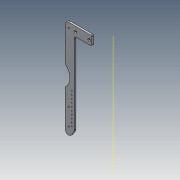
# Autodesk Inventor part: VP TRAY GUIDE SPLIT SHELF
Saved by Autodesk Inventor 2018.3 (Build 223284000, 284)
## iProperties
Created: 2018-09-09
Material: ACETAL COPOLYMER, WHITE
Vendor: HHMI: JRC - ID&F
Document SubType Name: Modeling
Designer: arnoldj
Density: 1.42 g/cm^3
Appearance: Plastic (White)
RuleStatus: InUse
AfterDocSave0: file://Part Number Cleaner
DESIGN DEPARTMENT: HHMI: JRC - ID&F
ALTERED ITEM PART NUMBER: N/A
ALTERED ITEM VENDOR: N/A
ALTERED ITEM DESCRIPTION: N/A
Author: arnoldj
Revision Number: 0
Autodesk Inventor part; units mm, degrees
ref_plane "YZ Plane" through (0, 0, 0) normal (1, 0, 0) x (0, 1, 0)
ref_plane "XZ Plane" through (0, 0, 0) normal (0, 1, 0) x (-1, 0, 0)
ref_plane "XY Plane" through (0, 0, 0) normal (0, 0, 1) x (1, 0, 0)
sketch "Sketch1" plane through (0, 0, 0) normal (0, 0, 1) x (1, 0, 0)
  line L0 (0, 251.46) -> (0, -264.16) projected
  line L1 (-361.3785, 0) -> (361.3785, 0) projected
  line L2 (177.8, -190.5) -> (-177.8, -190.5)
  line L3 (-177.8, -190.5) -> (-177.8, 177.8)
  line L4 (-177.8, 177.8) -> (177.8, 177.8)
  line L5 (177.8, 177.8) -> (177.8, -190.5)
  line L6 (143.51, -143.511) -> (-143.51, -143.511) construction
  line L7 (-143.51, -143.511) -> (-143.51, 143.509) construction
  line L8 (-143.51, 143.509) -> (143.51, 143.509) construction
  line L9 (143.51, 143.509) -> (143.51, -143.511) construction
  line L10 (-177.8, 177.8) -> (-177.8, 177.8)
  line L11 (-177.8, -190.5) -> (-177.8, 177.8)
  line L12 (177.8, 177.8) -> (177.8, 177.8)
  line L13 (177.8, -190.5) -> (177.8, 177.8)
  line L14 (-165.1, -158.75) -> (165.1, -158.75) construction
  line L15 (165.1, -158.75) -> (165.1, 158.75) construction
  line L16 (165.1, 158.75) -> (-165.1, 158.75) construction
  line L17 (-165.1, 158.75) -> (-165.1, -158.75) construction
  line L18 (144.4625, 143.509) -> (-144.4625, 143.509)
  line L19 (-144.4625, 143.509) -> (-144.4625, -190.5)
  line L20 (-144.4625, -190.5) -> (144.4625, -190.5)
  line L21 (144.4625, -190.5) -> (144.4625, 143.509)
  line L22 (144.4625, 143.509) -> (-144.4625, -190.5) construction
  line L23 (-144.4625, 143.509) -> (144.4625, -190.5) construction
  circle A0 centre (-209.55, 0) radius 48.5775
  circle A1 centre (209.55, 0) radius 48.5775
  line L24 (-65.455, 153.009) -> (-55.955, 153.009) construction
  line L25 (0, 177.8) -> (0, 143.509)
  point P0 (0, 0)
  point P1 (0, -23.4955)
  point P2 (-71.755, 153.009)
  point P3 (-139.7, 158.75)
  point P4 (139.7, 158.75)
  point P5 (0, 158.75)
  point P6 (-88.9, 158.75)
  point P7 (88.9, 158.75)
  point P8 (-165.1, -95.25)
  point P9 (165.1, -95.25)
  dimension "d2" = 355.6
  dimension "d66" = 177.8
  dimension "d70" = 368.3
  dimension "d71" = 177.8
  dimension "d85" = 287.02
  dimension "d86" = 330.2
  dimension "d94" = 288.925
  dimension "d95" = 0
  dimension "d107" = 209.55
  dimension "d108" = 97.155
  dimension "d111" = 209.55
  dimension "d112" = 9.5
  dimension "d113" = 9.5
  dimension "d115" = 15.8
  dimension "d116" = 71.755
  dimension "d124" = 139.7
  dimension "d125" = 139.7
  dimension "d133" = 317.5
  dimension "d134" = 165.1
  dimension "d135" = 158.75
  dimension "d136" = 50.8
  dimension "d137" = 50.8
  dimension "d158" = 63.5
  dimension "d159" = 63.5
  dimension "d160" = 55.955
  constraints: 48 end point, 12 point on line, 7 horizontal, 7 parallel, 5 coincident, 5 midpoint, 5 perpendicular, 2 centre point, 2 horizontal alignment, 1 equal radius
  measures "d2" distance of L3.end L4.end
  measures "d66" distance between parallel lines of L0 L3
  measures "d70" distance of L2.end L3.end
  measures "d71" distance between parallel lines of L1 L4
  measures "d85" distance of L6.end L7.end
  measures "d86" distance of L15.end L16.end
  measures "d94" distance of L18.start L18.end
  measures "d95" distance between parallel lines of L18 L8
  measures "d107" distance from line of L0 A0.centre
  measures "d108" diameter of A0
  measures "d111" distance from line of L0 A1.centre
  measures "d112" distance of L24.start L24.end
  measures "d113" distance between parallel lines of L24 L8
  measures "d115" distance of point (-55.955, 153.009) point (-71.755, 153.009)
  measures "d116" distance from line of L0 point (-71.755, 153.009)
  measures "d124" distance from line of point (-139.7, 158.75) L0
  measures "d125" distance from line of L0 point (139.7, 158.75)
  measures "d133" distance of L16.end L14.start
  measures "d134" distance between parallel lines of L0 L17
  measures "d135" distance between parallel lines of L1 L16
  measures "d136" distance of point (-139.7, 158.75) point (-88.9, 158.75)
  measures "d137" distance of point (88.9, 158.75) point (139.7, 158.75)
  measures "d158" distance from line of L14 point (-165.1, -95.25)
  measures "d159" distance of point (165.1, -95.25) point (165.1, -158.75)
  measures "d160" distance from line of L0 L24.end
extrude "Extrusion1" add sketch "Sketch1" against normal blind 6.35 contours L4 L5 A1 L1 L21 L18 L0 | L0 L18 L19 L1 A0 L3 L4 | L18 L21 L1 L0 | L0 L1 L19 L18 | L1 L21 L2 L0 | L0 L2 L19 L1 | A0 L1 L3 | L5 L1 A1 | L19 L2 L3 A0 L1 | L1 A1 L5 L2 L21 | L1 A0 L3 | L5 A1 L1 picked at (-175.8618, 22.522) picked at (175.8618, 22.522) picked at (-175.8618, -22.522) picked at (175.8618, -22.522)
hole "Hole5" at (-165.1, 158.75, 0) at (165.1, 158.75, 0) at (165.1, -158.75, 0) at (-165.1, -158.75, 0) at (-165.1, -95.25, 0) at (165.1, -95.25, 0) direction (0, 0, -1) diameter 5.1054 end through all clearance for "Flat Head Machine Screw (82)" size "#10" standard "Ansi Unified Screw Threads"
extrude "Extrusion5" cut sketch "Sketch1" against normal up to next contours L18 L21 L1 L0 | L0 L1 L19 L18 | L1 L21 L2 L0 | L0 L2 L19 L1
chamfer "Chamfer3" distance 15.875 angle 60 1 edges at (-144.4625, -190.5, -3.175) measured on face at (-166.6875, -190.5, -4.2333)
chamfer "Chamfer4" distance 15.875 angle 60 1 edges at (144.4625, -190.5, -3.175) measured on face at (155.575, -190.5, -4.2333)
fillet "Fillet8" radius 12.7 4 edges at (160.3375, -190.5, -3.175) (144.4625, -163.0037, -3.175) (-144.4625, -163.0037, -3.175) (-160.3375, -190.5, -3.175)
fillet "Fillet6" radius 12.7 4 edges at (177.8, -190.5, -3.175) (177.8, 177.8, -3.175) (-177.8, -190.5, -3.175) (-177.8, 177.8, -3.175)
fillet "Fillet7" radius 10.16 2 edges at (144.4625, 143.509, -3.175) (-144.4625, 143.509, -3.175)
extrude "Extrusion6" cut sketch "Sketch1" against normal up to next contours A0 L1 L3 | L3 L1 A0 | A1 L1 L5 | L5 L1 A1 | L3 A0 L1 | L1 A0 L3 | L5 A1 L1 | L1 A1 L5
hole "Hole6" at (-143.51, 143.509, 0) at (-65.455, 153.009, 0) at (-55.955, 153.009, 0) direction (0, 0, -1) diameter 1.524 end through all
mirror "Mirror1" about plane through (0, 0, 0) normal (1, 0, 0) of "Hole6"
hole "Hole7" at (-139.7, 158.75, 0) at (139.7, 158.75, 0) at (-88.9, 158.75, 0) at (88.9, 158.75, 0) direction (0, 0, -1) diameter 4.4958 end through all countersink diameter 9.398 countersink angle 90 clearance for "Flat Head Machine Screw" size "M4" standard "Ansi Metric M Profile"
sketch "Sketch3" plane through (0, 0, 0) normal (0, 0, 1) x (1, 0, 0)
  line L0 (0, 294.3121) -> (0, -274.6479) projected
  line L1 (-258.445, 0) -> (306.07, 0) projected
  line L2 (-79.375, 213.0321) -> (225.425, 213.0321)
  line L3 (225.425, 213.0321) -> (225.425, -193.3679)
  line L4 (225.425, -193.3679) -> (-79.375, -193.3679)
  line L5 (-79.375, -193.3679) -> (-79.375, 213.0321)
  line L6 (-177.8, -36.7656) -> (-177.8, -173.3489) projected
  line L7 (-144.4625, -159.6007) -> (-144.4625, 133.349) projected
  point P0 (0, 0)
  point P1 (-153.67, -152.4)
  dimension "d138" = 304.8
  dimension "d139" = 406.4
  dimension "d140" = 79.375
  dimension "d144" = 24.13
  dimension "d145" = 152.4
  dimension "d157" = 9.2075
  constraints: 8 end point, 2 parallel, 1 horizontal, 1 perpendicular
  measures "d138" distance of L2.start L2.end
  measures "d139" distance of L2.end L3.end
  measures "d140" distance between parallel lines of L0 L5
  measures "d144" distance from line of point (-153.67, -152.4) L6
  measures "d145" distance from line of point (-153.67, -152.4) L1
  measures "d157" distance from line of L7 point (-153.67, -152.4)
extrude "Extrusion7" cut sketch "Sketch3" against normal up to next
fillet "Fillet9" radius 3.175 2 edges at (-79.375, 143.509, -3.175) (-79.375, 177.8, -3.175)
hole "Hole8" at (-153.67, -152.4, 0) direction (0, 0, -1) diameter 3.2766 end through all clearance for "Flat Head Machine Screw (82)" size "#4" standard "Ansi Unified Screw Threads"
pattern_linear "Rectangular Pattern3" count 10 spacing 12.7 along (0, 1, 0) of "Hole8"
chamfer "Chamfer5" distance 2.4384 angle 45 2 edges at (-139.7, 160.9979, -6.35) (-88.9, 160.9979, -6.35)
ref_plane "Work Plane1" through (0, 0, 0) normal (1, 0, 0) x (0, 1, 0)
body "Solid1"
